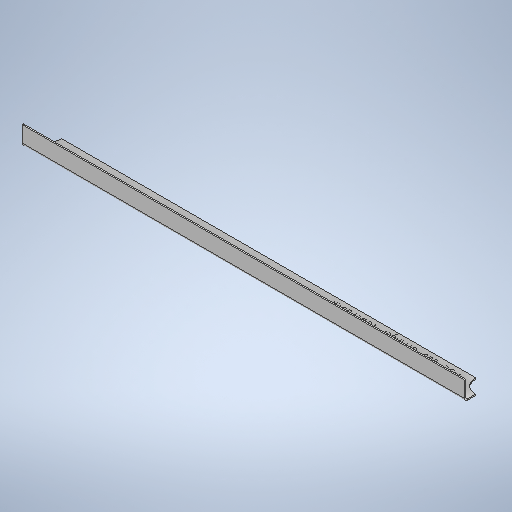
# Autodesk Inventor part: MSC 068 stringer lowerback
Saved by Autodesk Inventor 2025 (Build 290162010, 162A)
## iProperties
Created: 2024-04-28
Part Number: MSC 068 stringer lowerback
Material: Stainless Steel
Document SubType Name: Sheet Metal
Designer: admin
Stock Number: МОО 068 стрингер поясница
Density: 8 g/cm^3
Flat Pattern Width: 70 cm
Flat Pattern Length: 6.6202 cm
Flat Pattern Area: 463.414 cm^2
Sheet Metal Rule: AISI304 2mm Die16
Sheet Metal Width: 700,000 mm
Sheet Metal Length: 66,202 mm
Sheet Metal Area: 46341,393 mm^2
Appearance: Default
Author: admin
Autodesk Inventor part; units mm, degrees
ref_plane "YZ Plane" through (0, 0, 0) normal (1, 0, 0) x (0, 1, 0)
ref_plane "XZ Plane" through (0, 0, 0) normal (0, 1, 0) x (-1, 0, 0)
ref_plane "XY Plane" through (0, 0, 0) normal (0, 0, 1) x (1, 0, 0)
sketch "Sketch1" plane through (0, 0, 0) normal (0, 0, 1) x (1, 0, 0)
  line L0 (-700, 40) -> (0, 40)
  line L1 (0, 40) -> (0, 0)
  line L2 (0, 0) -> (-700, 0)
  line L3 (-700, 0) -> (-700, 40)
  point P0 (-350, 0)
  dimension "d1" = 40
  dimension "d45" = 700
  measures "d1" distance of L0.end L1.end
  measures "d45" distance of L1.end L2.end
extrude "Plate1" add sketch "Sketch1" along normal blind 2
sketch "Sketch2" plane through (0, 2, 0) normal (0, -1, 0) x (1, 0, 0)
  line L0 (-700, 0) -> (0, 0)
  line L1 (0, 0) -> (0, 30)
  line L2 (0, 30) -> (-700, 30)
  line L3 (-700, 30) -> (-700, 0)
  constraints: 6 end point, 1 horizontal, 1 perpendicular, 1 vertical
edge flange "Flange1" height 30 angle 90 thickness 2 bend radius 2.75 thickness toward (0, -1, 0) relief round relief width 2 relief depth 1 edges at (-350, 0, 2) wall of the first edge with corners at (-700, 2, 0) (0, 2, 0) (0, 2, 30) (-700, 2, 30)
bend "Bend1"
corner "Corner1"
sketch "Sketch6" plane through (0, 0, 0) normal (0, 0, -1) x (-1, 0, 0)
  line L0 (0, 40) -> (0, 4.75) projected
  circle A0 centre (0, 40) radius 22.5
  line L1 (0, 40) -> (700, 40) projected
  line L2 (-499, 30) -> (-499, 67.6691) projected
  point P0 (0, 0)
  point P1 (22.5, 40)
  point P2 (0, 17.5)
  dimension "d24" = 45
  constraints: 1 centre point, 1 other
  measures "d24" diameter of A0
extrude "Extrusion2" cut sketch "Sketch6" along normal mid plane 30 contours L1 A0 L0 picked at (14.812, 38.3311)
sketch "Sketch9" plane through (0, 0, 2) normal (0, 0, 1) x (1, 0, 0)
  line L0 (-38.0816, 35) -> (-38.0816, 23) construction
  line L1 (-38.0816, 23) -> (-238.0816, 23) construction
  line L2 (-238.0816, 23) -> (-238.0816, 35) construction
  line L3 (-238.0816, 35) -> (-38.0816, 35) construction
  line L4 (-700, 40) -> (0, 40) projected
  point P0 (0, 0)
  dimension "d40" = 200
  dimension "d41" = 12
  dimension "d43" = 5
  constraints: 2 other
  measures "d40" distance of L0.end L1.end
  measures "d41" distance of L1.end L2.end
  measures "d43" distance between parallel lines of L4 L3
mark "Mark2"
sketch "Sketch10" plane through (-700, 40, 2) normal (0, 0, 1) x (1, 0, 0)
  circle A0 centre (0, 0) radius 22.5
  line L0 (465.3629, -6.4882) -> (465.3629, -9.8215) projected
  line L1 (465.3629, -9.8215) -> (465.3629, -16.4882) projected
  line L2 (465.3629, -9.8215) -> (460.9184, -13.1549) projected
  line L3 (488.6962, -13.1549) -> (488.6962, -6.4882) projected
  line L4 (488.6962, -16.4882) -> (488.6962, -13.1549) projected
  line L5 (485.9184, -13.1549) -> (488.6962, -13.1549) projected
  arc A1 (484.2518, -11.4882) -> (485.9184, -13.1549) centre (485.9184, -11.4882) ccw projected
  line L6 (484.2518, -8.1549) -> (484.2518, -11.4882) projected
  arc A2 (485.9184, -6.4882) -> (484.2518, -8.1549) centre (485.9184, -8.1549) ccw projected
  line L7 (488.6962, -6.4882) -> (485.9184, -6.4882) projected
  line L8 (524.2518, -6.4882) -> (524.8073, -6.4882) projected
  arc A3 (526.474, -8.1549) -> (524.8073, -6.4882) centre (524.8073, -8.1549) ccw projected
  line L9 (526.474, -8.1549) -> (526.474, -16.4882) projected
  circle A4 centre (570.0851, -16.2104) radius 0.2778 projected
  line L10 (570.0851, -6.4882) -> (570.0851, -13.1549) projected
  line L11 (582.5851, -6.4882) -> (582.5851, -13.1549) projected
  line L12 (583.6962, -13.1549) -> (582.5851, -13.1549) projected
  line L13 (582.5851, -13.1549) -> (582.5851, -16.4882) projected
  line L14 (582.5851, -13.1549) -> (580.3629, -13.1549) projected
  line L15 (638.1407, -6.4882) -> (640.3629, -6.4882) projected
  arc A5 (642.5851, -8.7104) -> (640.3629, -6.4882) centre (640.3629, -8.7104) ccw projected
  line L16 (642.5851, -8.7104) -> (642.5851, -14.266) projected
  arc A6 (640.3629, -16.4882) -> (642.5851, -14.266) centre (640.3629, -14.266) ccw projected
  line L17 (640.3629, -16.4882) -> (638.1407, -16.4882) projected
  line L18 (660.9184, -6.4882) -> (660.9184, -16.4882) projected
  line L19 (660.9184, -16.4882) -> (657.5851, -10.9326) projected
  line L20 (657.5851, -10.9326) -> (654.2518, -16.4882) projected
  line L21 (654.2518, -16.4882) -> (654.2518, -6.4882) projected
  arc A7 (650.9184, -7.0437) -> (648.1407, -6.4882) centre (648.8513, -10.157) ccw projected
  arc A8 (648.1407, -6.4882) -> (647.0296, -10.9326) centre (648.2393, -8.874) ccw projected
  line L22 (647.0296, -10.9326) -> (649.8073, -12.5993) projected
  arc A9 (650.3629, -15.9326) -> (649.8073, -12.5993) centre (648.6785, -14.5004) ccw projected
  arc A10 (645.9184, -15.9326) -> (650.3629, -15.9326) centre (648.1407, -11.8029) ccw projected
  arc A11 (620.9184, -15.3771) -> (624.2518, -15.3771) centre (622.5851, -14.6897) ccw projected
  arc A12 (620.9184, -7.5993) -> (620.9184, -15.3771) centre (634.362, -11.4882) ccw projected
  arc A13 (624.2518, -7.5993) -> (620.9184, -7.5993) centre (622.5851, -8.308) ccw projected
  arc A14 (624.2518, -15.3771) -> (624.2518, -7.5993) centre (610.8082, -11.4882) ccw projected
  arc A15 (613.6962, -16.4882) -> (617.0296, -10.9326) centre (611.2666, -11.2526) ccw projected
  line L23 (617.0296, -10.9326) -> (617.0296, -8.7104) projected
  arc A16 (617.0296, -8.7104) -> (612.5851, -8.7104) centre (614.8073, -8.7104) ccw projected
  line L24 (612.5851, -8.7104) -> (612.5851, -9.8215) projected
  arc A17 (612.5851, -9.8215) -> (614.8073, -12.0437) centre (614.8073, -9.8215) ccw projected
  line L25 (614.8073, -12.0437) -> (616.474, -12.0437) projected
  line L26 (604.8073, -8.7104) -> (604.8073, -9.8215) projected
  arc A18 (609.2518, -8.7104) -> (604.8073, -8.7104) centre (607.0296, -8.7104) ccw projected
  line L27 (609.2518, -9.8215) -> (609.2518, -8.7104) projected
  arc A19 (607.0296, -12.0437) -> (609.2518, -9.8215) centre (607.0296, -9.8215) ccw projected
  line L28 (607.5851, -12.0437) -> (607.0296, -12.0437) projected
  arc A20 (609.2518, -13.7104) -> (607.5851, -12.0437) centre (607.5851, -13.7104) ccw projected
  line L29 (609.2518, -14.8215) -> (609.2518, -13.7104) projected
  arc A21 (607.5851, -16.4882) -> (609.2518, -14.8215) centre (607.5851, -14.8215) ccw projected
  line L30 (606.474, -16.4882) -> (607.5851, -16.4882) projected
  arc A22 (604.8073, -14.8215) -> (606.474, -16.4882) centre (606.474, -14.8215) ccw projected
  line L31 (604.8073, -13.7104) -> (604.8073, -14.8215) projected
  arc A23 (606.474, -12.0437) -> (604.8073, -13.7104) centre (606.474, -13.7104) ccw projected
  line L32 (607.0296, -12.0437) -> (606.474, -12.0437) projected
  arc A24 (604.8073, -9.8215) -> (607.0296, -12.0437) centre (607.0296, -9.8215) ccw projected
  arc A25 (591.474, -7.5993) -> (589.8073, -6.4882) centre (589.7954, -8.3116) ccw projected
  line L33 (589.8073, -6.4882) -> (588.6962, -6.4882) projected
  arc A26 (588.6962, -6.4882) -> (587.0296, -7.5993) centre (588.7081, -8.3116) ccw projected
  line L34 (587.0296, -7.5993) -> (587.0296, -8.1549) projected
  arc A27 (587.0296, -8.1549) -> (588.1407, -9.266) centre (588.8851, -7.4104) ccw projected
  line L35 (588.1407, -9.266) -> (590.3629, -10.3771) projected
  arc A28 (591.474, -11.4882) -> (590.3629, -10.3771) centre (589.6185, -12.2326) ccw projected
  line L36 (591.474, -11.4882) -> (591.474, -12.0437) projected
  arc A29 (589.8073, -13.1549) -> (591.474, -12.0437) centre (589.7954, -11.3314) ccw projected
  line L37 (589.8073, -13.1549) -> (588.6962, -13.1549) projected
  arc A30 (587.0296, -12.0437) -> (588.6962, -13.1549) centre (588.7081, -11.3314) ccw projected
  line L38 (577.0296, -6.4882) -> (577.0296, -13.1549) projected
  line L39 (577.0296, -13.1549) -> (574.8073, -13.1549) projected
  arc A31 (573.6962, -12.0437) -> (574.8073, -13.1549) centre (574.8073, -12.0437) ccw projected
  line L40 (566.474, -6.4882) -> (566.474, -13.1549) projected
  line L41 (566.474, -13.1549) -> (563.6962, -13.1549) projected
  arc A32 (562.0296, -11.4882) -> (563.6962, -13.1549) centre (563.6962, -11.4882) ccw projected
  line L42 (562.0296, -11.4882) -> (562.0296, -6.4882) projected
  line L43 (557.0296, -13.1549) -> (554.2518, -13.1549) projected
  line L44 (554.2518, -13.1549) -> (554.2518, -6.4882) projected
  line L45 (554.2518, -6.4882) -> (554.2518, -4.8215) projected
  arc A33 (555.9184, -3.1549) -> (554.2518, -4.8215) centre (555.9184, -4.8215) ccw projected
  line L46 (555.9184, -3.1549) -> (558.6962, -3.1549) projected
  line L47 (554.2518, -6.4882) -> (557.0296, -6.4882) projected
  arc A34 (558.6962, -8.1549) -> (557.0296, -6.4882) centre (557.0296, -8.1549) ccw projected
  line L48 (558.6962, -8.1549) -> (558.6962, -11.4882) projected
  arc A35 (557.0296, -13.1549) -> (558.6962, -11.4882) centre (557.0296, -11.4882) ccw projected
  line L49 (550.9184, -10.9326) -> (550.9184, -9.8215) projected
  arc A36 (546.474, -10.9326) -> (550.9184, -10.9326) centre (548.6962, -10.9326) ccw projected
  line L50 (546.474, -9.8215) -> (546.474, -10.9326) projected
  line L51 (550.9184, -9.8215) -> (546.474, -9.8215) projected
  line L52 (550.9184, -9.8215) -> (550.9184, -8.1549) projected
  arc A37 (550.9184, -8.1549) -> (549.2518, -6.4882) centre (549.2518, -8.1549) ccw projected
  line L53 (549.2518, -6.4882) -> (546.474, -6.4882) projected
  line L54 (543.1407, -6.4882) -> (543.1407, -13.1549) projected
  line L55 (543.1407, -13.1549) -> (540.9184, -13.1549) projected
  arc A38 (539.8073, -12.0437) -> (540.9184, -13.1549) centre (540.9184, -12.0437) ccw projected
  arc A39 (516.474, -10.9326) -> (520.9184, -10.9326) centre (518.6962, -10.9326) ccw projected
  line L56 (516.474, -8.7104) -> (516.474, -10.9326) projected
  arc A40 (520.9184, -8.7104) -> (516.474, -8.7104) centre (518.6962, -8.7104) ccw projected
  line L57 (520.9184, -10.9326) -> (520.9184, -8.7104) projected
  line L58 (513.1407, -13.1549) -> (511.474, -6.4882) projected
  line L59 (511.474, -6.4882) -> (509.8073, -10.9326) projected
  line L60 (509.8073, -10.9326) -> (508.1407, -6.4882) projected
  line L61 (508.1407, -6.4882) -> (506.474, -13.1549) projected
  line L62 (503.1407, -10.9326) -> (503.1407, -9.8215) projected
  arc A41 (498.6962, -10.9326) -> (503.1407, -10.9326) centre (500.9184, -10.9326) ccw projected
  line L63 (498.6962, -9.8215) -> (498.6962, -10.9326) projected
  line L64 (503.1407, -9.8215) -> (498.6962, -9.8215) projected
  line L65 (503.1407, -9.8215) -> (503.1407, -8.1549) projected
  arc A42 (503.1407, -8.1549) -> (501.474, -6.4882) centre (501.474, -8.1549) ccw projected
  line L66 (501.474, -6.4882) -> (498.6962, -6.4882) projected
  line L67 (495.3629, -6.4882) -> (495.3629, -13.1549) projected
  line L68 (495.3629, -13.1549) -> (493.1407, -13.1549) projected
  arc A43 (492.0296, -12.0437) -> (493.1407, -13.1549) centre (493.1407, -12.0437) ccw projected
  line L69 (478.6962, -13.1549) -> (476.474, -13.1549) projected
  line L70 (476.474, -13.1549) -> (476.474, -8.1549) projected
  line L71 (476.474, -8.1549) -> (476.474, -7.5993) projected
  arc A44 (476.474, -7.5993) -> (475.3629, -6.4882) centre (475.3629, -7.5993) ccw projected
  arc A45 (478.1407, -6.4882) -> (476.474, -8.1549) centre (478.1407, -8.1549) ccw projected
  line L72 (478.1407, -6.4882) -> (479.2518, -6.4882) projected
  arc A46 (480.9184, -8.1549) -> (479.2518, -6.4882) centre (479.2518, -8.1549) ccw projected
  line L73 (480.9184, -8.1549) -> (480.9184, -10.9326) projected
  arc A47 (478.6962, -13.1549) -> (480.9184, -10.9326) centre (478.6962, -10.9326) ccw projected
  line L74 (468.6962, -6.4882) -> (470.3629, -6.4882) projected
  arc A48 (472.0296, -8.1549) -> (470.3629, -6.4882) centre (470.3629, -8.1549) ccw projected
  line L75 (472.0296, -8.1549) -> (472.0296, -11.4882) projected
  arc A49 (470.3629, -13.1549) -> (472.0296, -11.4882) centre (470.3629, -11.4882) ccw projected
  line L76 (470.3629, -13.1549) -> (468.6962, -13.1549) projected
  line L77 (463.6962, -10.9326) -> (460.9184, -6.4882) projected
  arc A50 (677.5, 0) -> (700, -22.5) centre (700, 0) ccw projected
  line L78 (0, 0) -> (677.5, 0) projected
  line L79 (0, -35.25) -> (0, 0) projected
  line L80 (0, -35.25) -> (700, -35.25) projected
  line L81 (700, -22.5) -> (700, -35.25) projected
  point P0 (700, -40)
  point P1 (0, -22.5)
  point P2 (22.5, 0)
  dimension "d46" = 45
  constraints: 1 centre point, 1 coincident
  measures "d46" diameter of A0
extrude "Extrusion4" cut sketch "Sketch10" against normal through all contours A0 L79 L78 picked at (14.812, -1.6689)
equation "\"d43\" = d42"
equation "\"d2\" = Thickness"
equation "\"d3\" = BendReliefWidth"
equation "\"d4\" = BendReliefDepth"
equation "\"d5\" = MinimumRemnant"
equation "\"d6\" = TransitionRadius"
equation "\"d9\" = BendRadius"
equation "\"d10\" = CornerReliefSize"
equation "\"d11\" = GapSize"
equation "\"d12\" = JacobiRadiusSize"
equation "\"BendReliefWidth\" = Thickness"
equation "\"BendReliefDepth\" = 0.5 * Thickness"
equation "\"CornerReliefSize\" = 4 * Thickness"
equation "\"MinimumRemnant\" = 2 * Thickness"
equation "\"TransitionRadius\" = BendRadius"
equation "\"JacobiRadiusSize\" = BendRadius"
equation "\"GapSize\" = Thickness"
equation "\"qqqqqq\" = 67.35706"
equation "\"d42\" = 5"
equation "\"Thickness\" = 2"
equation "\"BendRadius\" = 2.75"
body "Solid1"
